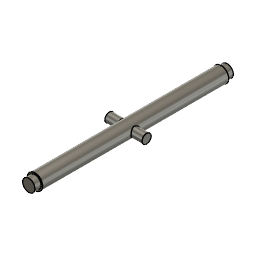
heatpipe (Autodesk Fusion 360 design; units mm, degrees)
part number: Configuration 3
Autodesk Fusion 360 part; units mm, degrees
sketch "Sketch8" plane through (0, 0, 0) normal (0, 0, 1) x (1, 0, 0)
  circle A0 centre (0, 0) radius 15
  circle A1 centre (0, 0) radius 25
  dimension "d21" = 30
  dimension "d22" = 50
  constraint coincident A0.centre A1.centre
  constraint concentric A0 A1
  measures "d21" diameter of A0
  measures "d22" diameter of A1
extrude "Extrude3" add sketch "Sketch8" along normal mid plane 600 makes body 1
sketch "Sketch9" plane through (0, 0, 0) normal (1, 0, 0) x (0, 0, -1)
  circle A0 centre (0, 0) radius 10
  circle A1 centre (0, 0) radius 15
  dimension "d25" = 20
  dimension "d26" = 30
  constraint coincident A0.centre A1.centre
  constraint concentric A0 A1
  measures "d25" diameter of A0
  measures "d26" diameter of A1
extrude "Extrude4" cut sketch "Sketch9" along normal mid plane 100 contours A0 bodies 1
extrude "Extrude5" add sketch "Sketch9" along normal mid plane 100 separate body makes body 2
extrude "Extrude6" cut sketch "Sketch8" along normal mid plane 600 contours A0 bodies 2
combine "Combine1" operation add target body 1 tool bodies 2
sketch "Sketch10" plane through (0, 0, -300) normal (0, 0, -1) x (-1, 0, 0)
  circle A0 centre (0, 0) radius 15
  circle A1 centre (0, 0) radius 25
  circle A2 centre (0, 0) radius 15
  circle A3 centre (0, 0) radius 20
  dimension "d33" = 30
  dimension "d34" = 40
  constraint concentric A0 A2
  constraint coincident A0.centre A1.centre
  measures "d33" diameter of A2
  measures "d34" diameter of A3
extrude "Extrude7" add sketch "Sketch10" along normal blind 10 contours A3 bodies 1
sketch "Sketch11" plane through (0, 0, 300) normal (0, 0, 1) x (1, 0, 0)
  circle A0 centre (0, 0) radius 15
  circle A1 centre (0, 0) radius 25
  circle A2 centre (0, 0) radius 15
  circle A3 centre (0, 0) radius 20
  dimension "d38" = 30
  dimension "d39" = 40
  constraint concentric A0 A2
  constraint concentric A2 A3
  measures "d38" diameter of A2
  measures "d39" diameter of A3
extrude "Extrude8" add sketch "Sketch11" along normal blind 10 contours A3 bodies 1
sketch "Sketch12" plane through (0, 0, -310) normal (0, 0, -1) x (-1, 0, 0)
  circle A0 centre (0, 0) radius 15
  circle A1 centre (0, 0) radius 20
  circle A2 centre (0, 0) radius 20
  dimension "d42" = 40
  constraint coincident A0.centre A1.centre
  measures "d42" diameter of A2
extrude "Extrude9" add sketch "Sketch12" along normal blind 10 contours A0 | A1 A2 bodies 1
sketch "Sketch13" plane through (0, 0, 310) normal (0, 0, 1) x (1, 0, 0)
  circle A0 centre (0, 0) radius 15
  circle A1 centre (0, 0) radius 20
  circle A2 centre (0, 0) radius 20
  dimension "d45" = 40
  constraint coincident A0.centre A1.centre
  measures "d45" diameter of A2
extrude "Extrude10" add sketch "Sketch13" along normal blind 10 contours A0 | A1 A2 bodies 1
sketch "Sketch14" plane through (-50, 0, 0) normal (-1, 0, 0) x (0, 0, 1)
  circle A0 centre (0, 0) radius 10
  circle A1 centre (0, 0) radius 15
  circle A2 centre (0, 0) radius 15
  dimension "d48" = 30
  constraint concentric A0 A2
  measures "d48" diameter of A2
extrude "Extrude11" add sketch "Sketch14" along normal blind 10 contours A0 | A1 A2 bodies 1
sketch "Sketch15" plane through (50, 0, 0) normal (1, 0, 0) x (0, 0, -1)
  circle A0 centre (0, 0) radius 10
  circle A1 centre (0, 0) radius 15
  circle A2 centre (0, 0) radius 15
  dimension "d51" = 30
  constraint coincident A0.centre A1.centre
  measures "d51" diameter of A2
extrude "Extrude12" add sketch "Sketch15" along normal blind 10 contours A0 | A1 A2 bodies 1
equation "LC_id = 30 mm" comment "Long Cylinder inner diameter"
equation "LC_od = 50 mm" comment "Long Cylinder outer diameter"
equation "SC_id = 20 mm" comment "Small arm Cylinder inner diameter"
equation "SC_od = 30 mm" comment "Small arm Cylinder outer diameter"
equation "LC_l = 300 mm" comment "Long Cylinder length"
equation "SC_l = 50 mm" comment "Short arm Cylinder length"
equation "SC_c = LC_l / 2.0" comment "Short arm Cylinder position (center of long cylinder length)"
equation "LC_w_id = LC_id" comment "lONG Cylinder cold window inner diameter"
equation "LC_w_od = 1.0 / 2.0 * ( LC_od + LC_id )" comment "Long Cylinder window outer diameter"
equation "d21 = LC_id"
equation "d22 = LC_od"
equation "d23 = LC_l"
equation "d25 = SC_id"
equation "d26 = SC_od"
equation "d27 = SC_l"
equation "d29 = SC_l"
equation "d31 = LC_l"
equation "d33 = LC_w_id"
equation "d34 = LC_w_od"
equation "LC_w_l = 10 mm" comment "Lenth of LC window cold tube"
equation "d36 = LC_w_l"
equation "d38 = LC_w_id"
equation "d39 = LC_w_od"
equation "d40 = LC_w_l"
equation "d42 = LC_w_od"
equation "d45 = LC_w_od"
equation "d48 = SC_od"
equation "d51 = SC_od"
